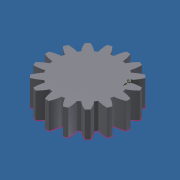
# Autodesk Inventor part: Stirnzahnrad2
Saved by Autodesk Inventor 2014 SP2 (Build 180246200, 246)
## iProperties
Created: 2014-12-13
Part Number: Stirnzahnrad2
Material: Steel
Document SubType Name: Modeling
Designer: 4ndreas
Categories: <?xml version="1.0" encoding="UTF-16"?> <MemberInstance><Categories><FamilyTemplate><FamilyTemplateParameter ValueType="xs:double" Id="1" ObjectReferenceKey="da_z" ObjectType="kUserParameterObject"/><FamilyTemplateParameter ValueType="xs:double" Id="2" ObjectReferenceKey="da_b" ObjectType="kUserParameterObject"/><FamilyTemplateParameter ValueType="xs:double" Id="3" ObjectReferenceKey="da_beta" ObjectType="kUserParameterObject"/><FamilyTemplateParameter ValueType="xs:double" Id="4" ObjectReferenceKey="da_da" ObjectType="kUserParameterObject"/><FamilyTemplateParameter ValueType="xs:double" Id="5" ObjectReferenceKey="da_aw" ObjectType="kUserParameterObject"/><FamilyTemplateParameter ValueType="xs:string" Id="6" ObjectReferenceKey="EAIAABAAAACIAQAAAAAAAIAAAAAAAAAA" ObjectType="83910656" SubObjectId="SurfaceGeometry"/></FamilyTemplate><ParamToTemplateMap><ParamToTemplate CategoryParameter="//CategoryParameter[@InternalName='046C89C9-8512-4d59-83FE-43B91F4F132A']" TemplateParameter="1"/><ParamToTemplate CategoryParameter="//CategoryParameter[@InternalName='2552DF32-E462-4b46-AEBF-C6C7768E72AC']" TemplateParameter="2"/><ParamToTemplate CategoryParameter="//CategoryParameter[@InternalName='C9EE641D-15FC-4fae-A226-E94C4372FDD7']" TemplateParameter="3"/><ParamToTemplate><ParamToTemplate CategoryParameter="//CategoryParameter[@InternalName='00B6519A-459B-49c7-AD84-2E56D39A5744']" ConstantValue="0.402671"/></ParamToTemplate><ParamToTemplate><ParamToTemplate CategoryParameter="//CategoryParameter[@InternalName='04B31F0E-C7A6-4894-AA32-9629BEFACF47']" ConstantValue="1.000000"/></ParamToTemplate><ParamToTemplate><ParamToTemplate CategoryParameter="//CategoryParameter[@InternalName='43CBEC2E-7847-49e7-A936-2F7889FCB2D9']" ConstantValue="0.250000"/></ParamToTemplate><ParamToTemplate><ParamToTemplate CategoryParameter="//CategoryParameter[@InternalName='B1EFC894-105D-4ebd-86BF-FA20ED196853']" ConstantValue="0.350000"/></ParamToTemplate><ParamToTemplate><ParamToTemplate CategoryParameter="//CategoryParameter[@InternalName='51175063-3D10-4879-93E8-6246FE8B403D']" ConstantValue="2060000000.000000"/></ParamToTemplate><ParamToTemplate><ParamToTemplate CategoryParameter="//CategoryParameter[@InternalName='A3A52E27-4454-46a9-B0BD-C932399B70AF']" ConstantValue="0.300000"/></ParamToTemplate><ParamToTemplate><ParamToTemplate CategoryParameter="//CategoryParameter[@InternalName='91B76062-C214-41d9-B1B9-14D2AB99603D']" ConstantValue="0.150000"/></ParamToTemplate><ParamToTemplate><ParamToTemplate CategoryParameter="//CategoryParameter[@InternalName='374E806E-8B8A-4dda-A9AA-1039D6500AD2']" ConstantValue="6.666667"/></ParamToTemplate><ParamToTemplate><ParamToTemplate CategoryParameter="//CategoryParameter[@InternalName='2D373A89-B862-43d6-8D0B-0CBF12AB9F6C']" ConstantValue="0.349066"/></ParamToTemplate><ParamToTemplate CategoryParameter="//CategoryParameter[@InternalName='37777632-D6A2-4fac-9D53-DB8ACD95C989']" TemplateParameter="4"/><ParamToTemplate CategoryParameter="//CategoryParameter[@InternalName='FD1017F1-B727-4f7e-9707-0F86F1FF9423']" TemplateParameter="5"/><ParamToTemplate><ParamToTemplate CategoryParameter="//CategoryParameter[@InternalName='9E1B4470-B2D3-4ff1-B813-535BB4CDF51A']" ConstantValue="3520000.000000"/></ParamToTemplate><ParamToTemplate><ParamToTemplate CategoryParameter="//CategoryParameter[@InternalName='F8452263-BFF6-458c-9FB1-07C4B99E95CD']" ConstantValue="11400000.000000"/></ParamToTemplate><ParamToTemplate><ParamToTemplate CategoryParameter="//CategoryParameter[@InternalName='3E3BB259-FD49-497f-8171-6EBC954A3479']" ConstantValue="2.000000"/></ParamToTemplate><ParamToTemplate CategoryParameter="//CategoryParameter[@InternalName='27C3BAF2-7550-4e4b-AE2C-0DB134B7D9B7']" TemplateParameter="6"/></ParamToTemplateMap><Category DisplayName="Gear" InternalName="DC85795E-93AB-48d5-8EEE-5A27447B64BD" Mnemonic="Gear"><CategoryParameter DisplayName="z" InternalName="046C89C9-8512-4d59-83FE-43B91F4F132A" Mnemonic="z"/><CategoryParameter DisplayName="b" InternalName="2552DF32-E462-4b46-AEBF-C6C7768E72AC" Mnemonic="b"/><CategoryParameter DisplayName="||b|" InternalName="C9EE641D-15FC-4fae-A226-E94C4372FDD7" Mnemonic="beta"/><CategoryParameter DisplayName="x" InternalName="00B6519A-459B-49c7-AD84-2E56D39A5744" Mnemonic="x"/><CategoryParameter DisplayName="a*" InternalName="04B31F0E-C7A6-4894-AA32-9629BEFACF47" Mnemonic="a"/><CategoryParameter DisplayName="c*" InternalName="43CBEC2E-7847-49e7-A936-2F7889FCB2D9" Mnemonic="c"/><CategoryParameter DisplayName="r|.f|*" InternalName="B1EFC894-105D-4ebd-86BF-FA20ED196853" Mnemonic="rf"/><CategoryParameter DisplayName="E" InternalName="51175063-3D10-4879-93E8-6246FE8B403D" Mnemonic="E"/><CategoryParameter DisplayName="||m|" InternalName="A3A52E27-4454-46a9-B0BD-C932399B70AF" Mnemonic="mi"/><Category DisplayName="SpurGear" InternalName="26C5A22E-A91E-4dfd-A3B3-23CCAFAE1764" Mnemonic="SpurGear"><CategoryParameter DisplayName="m" InternalName="91B76062-C214-41d9-B1B9-14D2AB99603D" Mnemonic="m"/><CategoryParameter DisplayName="P" InternalName="374E806E-8B8A-4dda-A9AA-1039D6500AD2" Mnemonic="PP"/><CategoryParameter DisplayName="||a|" InternalName="2D373A89-B862-43d6-8D0B-0CBF12AB9F6C" Mnemonic="alpha"/><CategoryParameter DisplayName="d|.a|" InternalName="37777632-D6A2-4fac-9D53-DB8ACD95C989" Mnemonic="da"/><CategoryParameter DisplayName="a|.w|" InternalName="FD1017F1-B727-4f7e-9707-0F86F1FF9423" Mnemonic="aw"/><CategoryParameter DisplayName="||s||.Flim|" InternalName="9E1B4470-B2D3-4ff1-B813-535BB4CDF51A" Mnemonic="sFlim"/><CategoryParameter DisplayName="||s||.Hlim|" InternalName="F8452263-BFF6-458c-9FB1-07C4B99E95CD" Mnemonic="sHlim"/><CategoryParameter DisplayName="Typ" InternalName="3E3BB259-FD49-497f-8171-6EBC954A3479" Mnemonic="type"/><CategoryParameter DisplayName="PitchDiameter" InternalName="27C3BAF2-7550-4e4b-AE2C-0DB134B7D9B7" Mnemonic="IDS_PITCHDIAM"/></Category></Category></Categories></MemberInstance>
Density: 1 g/cm^3
Appearance: Steel
CustomPartVersion: 1
Author: 4ndreas
Autodesk Inventor part; units mm, degrees
sketch "Sketch1" plane through (0, 0, 0) normal (0, 0, 1) x (1, 0, 0)
  circle A0 centre (0, 0) radius 14.104
  dimension "d0" = 28.208
  constraints: 1 centre point
  measures "d0" diameter of A0
extrude "Extrusion1" add sketch "Sketch1" along normal blind 9
ref_plane "Work Plane2" through (0, 0, 4.5) normal (0, 0, 1) x (1, 0, 0)
sketch "Sketch2" plane through (0, 0, 0) normal (0, 0, -1) x (-1, 0, 0)
  circle A0 centre (0, 0) radius 14.104 projected
  circle A1 centre (0, 0) radius 11.8406
  dimension "d3" = 23.6812
  constraints: 1 centre point, 1 coincident
  measures "d3" diameter of A1
surface extrude "Flankendurchmesser" sketch "Sketch2" against normal through all shown no curves A1
ref_plane "Work Plane8" through (0, 0, 0) normal (0.9807853, 0.1950903, 0) x (0, 0, 1)
ref_plane "Work Plane9" through (0, 0, 0) normal (1, 0, 0) x (0, 1, 0)
spur gear teeth "Stirnzahnrad" teeth 16 pitch diameter 24 tip diameter 28.208 root diameter 21.458 face width 9 start plane through (0, 0, 0) normal (0, 0, -1) x (-1, 0, 0)
sketch "Skizze3" plane through (0, 0, 0) normal (0, 0, -1) x (-1, 0, 0)
  arc A0 (5.5158, 9.2026) -> (6.0302, 12.7499) centre (-4.9001, 12.524) ccw projected
  arc A1 (6.0302, 12.7499) -> (4.7515, 13.2795) centre (0, 0) ccw projected
  arc A2 (4.7515, 13.2795) -> (2.6069, 10.4075) centre (12.3207, 5.3909) ccw projected
  arc A3 (2.6069, 10.4075) -> (1.5743, 10.6129) centre (0, 0) ccw projected
  arc A4 (1.5743, 10.6129) -> (0.6921, 14.087) centre (-9.3199, 9.6955) ccw projected
  arc A5 (0.6921, 14.087) -> (-0.6921, 14.087) centre (0, 0) ccw projected
  arc A6 (-0.6921, 14.087) -> (-1.5743, 10.6129) centre (9.3199, 9.6955) ccw projected
  arc A7 (-1.5743, 10.6129) -> (-2.6069, 10.4075) centre (0, 0) ccw projected
  arc A8 (-2.6069, 10.4075) -> (-4.7515, 13.2795) centre (-12.3207, 5.3909) ccw projected
  arc A9 (-4.7515, 13.2795) -> (-6.0302, 12.7499) centre (0, 0) ccw projected
  arc A10 (-6.0302, 12.7499) -> (-5.5158, 9.2026) centre (4.9001, 12.524) ccw projected
  arc A11 (-5.5158, 9.2026) -> (-6.3913, 8.6176) centre (0, 0) ccw projected
  arc A12 (-6.3913, 8.6176) -> (-9.4717, 10.4504) centre (-13.4459, 0.2656) ccw projected
  arc A13 (-9.4717, 10.4504) -> (-10.4504, 9.4717) centre (0, 0) ccw projected
  arc A14 (-10.4504, 9.4717) -> (-8.6176, 6.3913) centre (-0.2656, 13.4459) ccw projected
  arc A15 (-8.6176, 6.3913) -> (-9.2026, 5.5158) centre (0, 0) ccw projected
  arc A16 (-9.2026, 5.5158) -> (-12.7499, 6.0302) centre (-12.524, -4.9001) ccw projected
  arc A17 (-12.7499, 6.0302) -> (-13.2795, 4.7515) centre (0, 0) ccw projected
  arc A18 (-13.2795, 4.7515) -> (-10.4075, 2.6069) centre (-5.3909, 12.3207) ccw projected
  arc A19 (-10.4075, 2.6069) -> (-10.6129, 1.5743) centre (0, 0) ccw projected
  arc A20 (-10.6129, 1.5743) -> (-14.087, 0.6921) centre (-9.6955, -9.3199) ccw projected
  arc A21 (-14.087, 0.6921) -> (-14.087, -0.6921) centre (0, 0) ccw projected
  arc A22 (-14.087, -0.6921) -> (-10.6129, -1.5743) centre (-9.6955, 9.3199) ccw projected
  arc A23 (-10.6129, -1.5743) -> (-10.4075, -2.6069) centre (0, 0) ccw projected
  arc A24 (-10.4075, -2.6069) -> (-13.2795, -4.7515) centre (-5.3909, -12.3207) ccw projected
  arc A25 (-13.2795, -4.7515) -> (-12.7499, -6.0302) centre (0, 0) ccw projected
  arc A26 (-12.7499, -6.0302) -> (-9.2026, -5.5158) centre (-12.524, 4.9001) ccw projected
  arc A27 (-9.2026, -5.5158) -> (-8.6176, -6.3913) centre (0, 0) ccw projected
  arc A28 (-8.6176, -6.3913) -> (-10.4504, -9.4717) centre (-0.2656, -13.4459) ccw projected
  arc A29 (-10.4504, -9.4717) -> (-9.4717, -10.4504) centre (0, 0) ccw projected
  arc A30 (-9.4717, -10.4504) -> (-6.3913, -8.6176) centre (-13.4459, -0.2656) ccw projected
  arc A31 (-6.3913, -8.6176) -> (-5.5158, -9.2026) centre (0, 0) ccw projected
  arc A32 (-5.5158, -9.2026) -> (-6.0302, -12.7499) centre (4.9001, -12.524) ccw projected
  arc A33 (-6.0302, -12.7499) -> (-4.7515, -13.2795) centre (0, 0) ccw projected
  arc A34 (-4.7515, -13.2795) -> (-2.6069, -10.4075) centre (-12.3207, -5.3909) ccw projected
  arc A35 (-2.6069, -10.4075) -> (-1.5743, -10.6129) centre (0, 0) ccw projected
  arc A36 (-1.5743, -10.6129) -> (-0.6921, -14.087) centre (9.3199, -9.6955) ccw projected
  arc A37 (-0.6921, -14.087) -> (0.6921, -14.087) centre (0, 0) ccw projected
  arc A38 (0.6921, -14.087) -> (1.5743, -10.6129) centre (-9.3199, -9.6955) ccw projected
  arc A39 (1.5743, -10.6129) -> (2.6069, -10.4075) centre (0, 0) ccw projected
  arc A40 (2.6069, -10.4075) -> (4.7515, -13.2795) centre (12.3207, -5.3909) ccw projected
  arc A41 (4.7515, -13.2795) -> (6.0302, -12.7499) centre (0, 0) ccw projected
  arc A42 (6.0302, -12.7499) -> (5.5158, -9.2026) centre (-4.9001, -12.524) ccw projected
  arc A43 (5.5158, -9.2026) -> (6.3913, -8.6176) centre (0, 0) ccw projected
  arc A44 (6.3913, -8.6176) -> (9.4717, -10.4504) centre (13.4459, -0.2656) ccw projected
  arc A45 (9.4717, -10.4504) -> (10.4504, -9.4717) centre (0, 0) ccw projected
  arc A46 (10.4504, -9.4717) -> (8.6176, -6.3913) centre (0.2656, -13.4459) ccw projected
  arc A47 (8.6176, -6.3913) -> (9.2026, -5.5158) centre (0, 0) ccw projected
  arc A48 (9.2026, -5.5158) -> (12.7499, -6.0302) centre (12.524, 4.9001) ccw projected
  arc A49 (12.7499, -6.0302) -> (13.2795, -4.7515) centre (0, 0) ccw projected
  arc A50 (13.2795, -4.7515) -> (10.4075, -2.6069) centre (5.3909, -12.3207) ccw projected
  arc A51 (10.4075, -2.6069) -> (10.6129, -1.5743) centre (0, 0) ccw projected
  arc A52 (10.6129, -1.5743) -> (14.087, -0.6921) centre (9.6955, 9.3199) ccw projected
  arc A53 (14.087, -0.6921) -> (14.087, 0.6921) centre (0, 0) ccw projected
  arc A54 (14.087, 0.6921) -> (10.6129, 1.5743) centre (9.6955, -9.3199) ccw projected
  arc A55 (10.6129, 1.5743) -> (10.4075, 2.6069) centre (0, 0) ccw projected
  arc A56 (10.4075, 2.6069) -> (13.2795, 4.7515) centre (5.3909, 12.3207) ccw projected
  arc A57 (13.2795, 4.7515) -> (12.7499, 6.0302) centre (0, 0) ccw projected
  arc A58 (12.7499, 6.0302) -> (9.2026, 5.5158) centre (12.524, -4.9001) ccw projected
  arc A59 (9.2026, 5.5158) -> (8.6176, 6.3913) centre (0, 0) ccw projected
  arc A60 (8.6176, 6.3913) -> (10.4504, 9.4717) centre (0.2656, 13.4459) ccw projected
  arc A61 (10.4504, 9.4717) -> (9.4717, 10.4504) centre (0, 0) ccw projected
  arc A62 (9.4717, 10.4504) -> (6.3913, 8.6176) centre (13.4459, 0.2656) ccw projected
  arc A63 (6.3913, 8.6176) -> (5.5158, 9.2026) centre (0, 0) ccw projected
  arc A64 (0.5581, 13.8928) -> (-0.5581, 13.8928) centre (0, 0) ccw
  arc A65 (1.3872, 10.4372) -> (0.5581, 13.8928) centre (-9.3199, 9.6955) ccw
  arc A66 (2.7126, 10.1736) -> (1.3872, 10.4372) centre (0, 0) ccw
  arc A67 (4.801, 13.0488) -> (2.7126, 10.1736) centre (12.3207, 5.3909) ccw
  arc A68 (5.8321, 12.6217) -> (4.801, 13.0488) centre (0, 0) ccw
  arc A69 (5.2757, 9.1119) -> (5.8321, 12.6217) centre (-4.9001, 12.524) ccw
  arc A70 (6.3994, 8.3611) -> (5.2757, 9.1119) centre (0, 0) ccw
  arc A71 (9.4291, 10.2183) -> (6.3994, 8.3611) centre (13.4459, 0.2656) ccw
  arc A72 (10.2183, 9.4291) -> (9.4291, 10.2183) centre (0, 0) ccw
  arc A73 (8.3611, 6.3994) -> (10.2183, 9.4291) centre (0.2656, 13.4459) ccw
  arc A74 (9.1119, 5.2757) -> (8.3611, 6.3994) centre (0, 0) ccw
  arc A75 (12.6217, 5.8321) -> (9.1119, 5.2757) centre (12.524, -4.9001) ccw
  arc A76 (13.0488, 4.801) -> (12.6217, 5.8321) centre (0, 0) ccw
  arc A77 (10.1736, 2.7126) -> (13.0488, 4.801) centre (5.3909, 12.3207) ccw
  arc A78 (10.4372, 1.3872) -> (10.1736, 2.7126) centre (0, 0) ccw
  arc A79 (13.8928, 0.5581) -> (10.4372, 1.3872) centre (9.6955, -9.3199) ccw
  arc A80 (13.8928, -0.5581) -> (13.8928, 0.5581) centre (0, 0) ccw
  arc A81 (10.4372, -1.3872) -> (13.8928, -0.5581) centre (9.6955, 9.3199) ccw
  arc A82 (10.1736, -2.7126) -> (10.4372, -1.3872) centre (0, 0) ccw
  arc A83 (13.0488, -4.801) -> (10.1736, -2.7126) centre (5.3909, -12.3207) ccw
  arc A84 (12.6217, -5.8321) -> (13.0488, -4.801) centre (0, 0) ccw
  arc A85 (9.1119, -5.2757) -> (12.6217, -5.8321) centre (12.524, 4.9001) ccw
  arc A86 (8.3611, -6.3994) -> (9.1119, -5.2757) centre (0, 0) ccw
  arc A87 (10.2183, -9.4291) -> (8.3611, -6.3994) centre (0.2656, -13.4459) ccw
  arc A88 (9.4291, -10.2183) -> (10.2183, -9.4291) centre (0, 0) ccw
  arc A89 (6.3994, -8.3611) -> (9.4291, -10.2183) centre (13.4459, -0.2656) ccw
  arc A90 (5.2757, -9.1119) -> (6.3994, -8.3611) centre (0, 0) ccw
  arc A91 (5.8321, -12.6217) -> (5.2757, -9.1119) centre (-4.9001, -12.524) ccw
  arc A92 (4.801, -13.0488) -> (5.8321, -12.6217) centre (0, 0) ccw
  arc A93 (2.7126, -10.1736) -> (4.801, -13.0488) centre (12.3207, -5.3909) ccw
  arc A94 (1.3872, -10.4372) -> (2.7126, -10.1736) centre (0, 0) ccw
  arc A95 (0.5581, -13.8928) -> (1.3872, -10.4372) centre (-9.3199, -9.6955) ccw
  arc A96 (-0.5581, -13.8928) -> (0.5581, -13.8928) centre (0, 0) ccw
  arc A97 (-1.3872, -10.4372) -> (-0.5581, -13.8928) centre (9.3199, -9.6955) ccw
  arc A98 (-2.7126, -10.1736) -> (-1.3872, -10.4372) centre (0, 0) ccw
  arc A99 (-4.801, -13.0488) -> (-2.7126, -10.1736) centre (-12.3207, -5.3909) ccw
  arc A100 (-5.8321, -12.6217) -> (-4.801, -13.0488) centre (0, 0) ccw
  arc A101 (-5.2757, -9.1119) -> (-5.8321, -12.6217) centre (4.9001, -12.524) ccw
  arc A102 (-6.3994, -8.3611) -> (-5.2757, -9.1119) centre (0, 0) ccw
  arc A103 (-9.4291, -10.2183) -> (-6.3994, -8.3611) centre (-13.4459, -0.2656) ccw
  arc A104 (-10.2183, -9.4291) -> (-9.4291, -10.2183) centre (0, 0) ccw
  arc A105 (-8.3611, -6.3994) -> (-10.2183, -9.4291) centre (-0.2656, -13.4459) ccw
  arc A106 (-9.1119, -5.2757) -> (-8.3611, -6.3994) centre (0, 0) ccw
  arc A107 (-12.6217, -5.8321) -> (-9.1119, -5.2757) centre (-12.524, 4.9001) ccw
  arc A108 (-13.0488, -4.801) -> (-12.6217, -5.8321) centre (0, 0) ccw
  arc A109 (-10.1736, -2.7126) -> (-13.0488, -4.801) centre (-5.3909, -12.3207) ccw
  arc A110 (-10.4372, -1.3872) -> (-10.1736, -2.7126) centre (0, 0) ccw
  arc A111 (-13.8928, -0.5581) -> (-10.4372, -1.3872) centre (-9.6955, 9.3199) ccw
  arc A112 (-13.8928, 0.5581) -> (-13.8928, -0.5581) centre (0, 0) ccw
  arc A113 (-10.4372, 1.3872) -> (-13.8928, 0.5581) centre (-9.6955, -9.3199) ccw
  arc A114 (-10.1736, 2.7126) -> (-10.4372, 1.3872) centre (0, 0) ccw
  arc A115 (-13.0488, 4.801) -> (-10.1736, 2.7126) centre (-5.3909, 12.3207) ccw
  arc A116 (-12.6217, 5.8321) -> (-13.0488, 4.801) centre (0, 0) ccw
  arc A117 (-9.1119, 5.2757) -> (-12.6217, 5.8321) centre (-12.524, -4.9001) ccw
  arc A118 (-8.3611, 6.3994) -> (-9.1119, 5.2757) centre (0, 0) ccw
  arc A119 (-10.2183, 9.4291) -> (-8.3611, 6.3994) centre (-0.2656, 13.4459) ccw
  arc A120 (-9.4291, 10.2183) -> (-10.2183, 9.4291) centre (0, 0) ccw
  arc A121 (-6.3994, 8.3611) -> (-9.4291, 10.2183) centre (-13.4459, 0.2656) ccw
  arc A122 (-5.2757, 9.1119) -> (-6.3994, 8.3611) centre (0, 0) ccw
  arc A123 (-5.8321, 12.6217) -> (-5.2757, 9.1119) centre (4.9001, 12.524) ccw
  arc A124 (-4.801, 13.0488) -> (-5.8321, 12.6217) centre (0, 0) ccw
  arc A125 (-2.7126, 10.1736) -> (-4.801, 13.0488) centre (-12.3207, 5.3909) ccw
  arc A126 (-1.3872, 10.4372) -> (-2.7126, 10.1736) centre (0, 0) ccw
  arc A127 (-0.5581, 13.8928) -> (-1.3872, 10.4372) centre (9.3199, 9.6955) ccw
  dimension "d49" = 0.2
  constraints: 128 point on circle, 64 centre point, 63 other
  measures "d49" radial gap between concentric circles of A64 A5
equation "\"d0\" = da_da"
equation "\"d1\" = da_b"
equation "\"d3\" = da_dw"
equation "\"d16\" = da_aw"
equation "\"d43\" = da_aw"
equation "\"d46\" = da_aw"
equation "\"da_da\" = 28.208013"
equation "\"da_b\" = 9"
equation "\"da_dw\" = 23.681201"
equation "\"da_aw\" = 47.362402"
body "Solid1"
body "Srf1"
